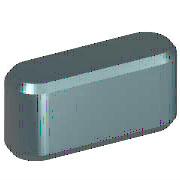
# Autodesk Inventor part: 键 GB/T 1566 A14 x 6 x 40
Saved by Autodesk Inventor 2025 (Build 290162000, 162)
## iProperties
Created: 2024-01-20
Part Number: 键 GB/T 1566 A14 x 6 x 40
Material: 钢，软
Description: 方形和矩形窄键槽
Document SubType Name: Modeling
Standard: GB/T 1566-2003
Designer: ASUS
Standard Revision: 2003
Standards Organization: GB
Language: zh-CN
Size Designation: A - 14 x 6 x 40
Categories: <MemberInstance><Categories><Category DisplayName="轴用零件" InternalName="7f7aeb1f-a693-4053-b835-cee3144e0d98" Mnemonic="SHFT"><Category DisplayName="键" InternalName="7048e72f-fdca-4e3b-88b7-55969eb6630e" Mnemonic="KEY"><CategoryParameter DisplayName="宽度" InternalName="34be0dd5-dba5-4911-b4ec-c22f2bfaa692" Mnemonic="kwdth"/><CategoryParameter DisplayName="最大轴肩直径" InternalName="95a81a26-4bdb-43e8-b886-6e2d08494928" Mnemonic="maxshdia"/><CategoryParameter DisplayName="最小轴肩直径" InternalName="b06394f3-cee7-4e5b-902c-663fb38acff4" Mnemonic="minshdia"/><CategoryParameter DisplayName="尺寸" InternalName="da4729c0-75a4-4053-9158-804a4a937d72" Mnemonic="keysize"/><CategoryParameter DisplayName="轴直径范围 (最小 - 最大)" InternalName="e5432c95-44d4-4c4b-a96d-eed0500887aa" Mnemonic="shaftdiarng"/><CategoryParameter DisplayName="轴直径" InternalName="ff971ec2-6a20-455a-900e-83f11d6bc337" Mnemonic="shaftdia"/><Category DisplayName="键 - 机制" InternalName="7a219f9c-bd0a-4811-91fb-2e47d97adffa" Mnemonic="PRLKEY"><CategoryParameter DisplayName="类型" InternalName="16552a72-3a79-47b2-9cce-0bdb5ab712ec" Mnemonic="keytype"/><CategoryParameter DisplayName="长度" InternalName="2aaf8abc-e798-4f7a-b8d4-83df963ddd80" Mnemonic="klen"/><CategoryParameter DisplayName="平键槽深" InternalName="b2aecbbc-9c00-4ee8-a417-d7ce8bca5723" Mnemonic="groovedepth"/><CategoryParameter DisplayName="高度" InternalName="d0342fb0-ff3c-42cf-83d6-cbe58e85d3e8" Mnemonic="kheig"/><CategoryParameter DisplayName="键槽深" InternalName="e370d4da-8754-4912-963a-6e35f2b6573a" Mnemonic="hubdepth"/><Category DisplayName="圆形" InternalName="c65a28b4-1924-4107-97a1-2d8922e9707a" Mnemonic="PRLKEYROUND"/></Category></Category></Category><Category DisplayName="数据类型" InternalName="23b78d0f-2648-40c6-8793-ca6db495c9e8" Mnemonic="DATATYPE"><CategoryParameter DisplayName="显示名" InternalName="05415f3d-3907-474b-a020-eb9d644f4cf3" Mnemonic="DISPLAYNAME"/><CategoryParameter DisplayName="标准" InternalName="0c0a119c-1e12-4c84-803f-101930972f5e" Mnemonic="STANDARD"/><CategoryParameter DisplayName="描述" InternalName="13903e3d-64b1-4950-80da-f627842ea37f" Mnemonic="DESCRIPTION"/><CategoryParameter DisplayName="规格" InternalName="2675968c-4ce5-49e0-a4f5-552d29089031" Mnemonic="DESIGNATION"/><CategoryParameter DisplayName="默认列" InternalName="2af9ec52-faaa-4026-b378-f9fa4afca842" Mnemonic="DEFAULTROW"/><CategoryParameter DisplayName="文件夹名称" InternalName="3f06958e-8713-4116-9be7-ed6184ecc97b" Mnemonic="FOLDERNAME"/><CategoryParameter DisplayName="版本指南" InternalName="45a75005-10b1-4dfc-8d6d-dfe629f0b93c" Mnemonic="REVISIONGUID"/><CategoryParameter DisplayName="文件名" InternalName="8b46a4cc-9585-4fed-90c3-899f57e09a73" Mnemonic="FILENAME"/><CategoryParameter DisplayName="标准组织" InternalName="8f5914e1-4693-403f-8ab5-d37768198c9d" Mnemonic="STDSORG"/><CategoryParameter DisplayName="系列版本" InternalName="914462f6-6e19-4b14-ba84-155b9680b1d0" Mnemonic="FAMILYREVISION"/><CategoryParameter DisplayName="标准版本" InternalName="91d5a463-65c2-4fde-b823-3b7fea5e8e17" Mnemonic="STANDARDREVISION"/><CategoryParameter DisplayName="成员版本" InternalName="a65d44b9-392f-4f4f-857b-e4b3d54996fe" Mnemonic="MEMBERREVISION"/><CategoryParameter DisplayName="剪裁格式" InternalName="bc51e27b-3422-4e78-93ef-cec197ddf230" Mnemonic="CLIPFORMAT"/><CategoryParameter DisplayName="制造商" InternalName="cd6c7a72-a28a-4e50-99a9-2c7f4e13e5ad" Mnemonic="MANUFACTURER"/><CategoryParameter DisplayName="内部名称" InternalName="cf1d0246-76d9-4b4a-8305-fa0409afb5c1" Mnemonic="INTERNALNAME"/><CategoryParameter DisplayName="是否公制" InternalName="e2385c5b-1ea4-4823-96a8-8de651266ec3" Mnemonic="ISMETRIC"/><Category DisplayName="零件" InternalName="c0e0b642-3bcb-4cc8-9e80-f96d35c4afa4" Mnemonic="PART"><CategoryParameter DisplayName="零件代号" InternalName="016b6077-bfbe-49bd-92c9-d8d59c39c941" Mnemonic="PARTNUMBER"/><CategoryParameter DisplayName="库存编号" InternalName="4dba7c1c-e26c-444e-836c-b08b433409a8" Mnemonic="STOCKNUMBER"/><CategoryParameter DisplayName="材料键" InternalName="5c9a8adb-dd2b-4535-b97f-0a94a95fe41f" Mnemonic="MATERIALKEY"/><CategoryParameter DisplayName="材料" InternalName="818a152a-d3c3-49ca-80ee-df7d91421b8e" Mnemonic="MATERIAL"/></Category></Category><Category DisplayName="先前版本映射" InternalName="cd87c42b-3e48-431e-b5c0-1cbeb14dfe77" Mnemonic="LEGACYMAP"><CategoryParameter DisplayName="唯一 DA 成员 ID" InternalName="0918ad47-427f-4fed-ae26-24c81c58f590" Mnemonic="DACOOKIE"/><CategoryParameter DisplayName="合并11 ID" InternalName="0ee8fb18-e2ed-4f39-96f6-1f4b5f50aa71" Mnemonic="MERGE11"/><CategoryParameter DisplayName="唯一 CC 成员 ID" InternalName="5193edd4-b2b0-4ab4-9d54-de900eee34e0" Mnemonic="CCCOOKIE"/><CategoryParameter DisplayName="分割 ID" InternalName="72b5c83c-be7f-45c4-ae51-9160ea6deb26" Mnemonic="SPLIT"/><CategoryParameter DisplayName="成员 ID" InternalName="8e5e0294-fc51-4c8f-b3d7-003dc5ed94f6" Mnemonic="MEMBERID"/><CategoryParameter DisplayName="目录名" InternalName="d99d1e27-aa94-4de2-af4c-c348882a6f4f" Mnemonic="CATALOGNAME"/><CategoryParameter DisplayName="系列编号" InternalName="e705e1f4-09cb-413e-91f9-551b4188271e" Mnemonic="FAMILYNUMBER"/></Category></Categories><FamilyTemplate Id="si0114"><FamilyTemplateParameters><FamilyTemplateParameter ObjectType="kUserParameterObject" ValueType="xs:double" Id="1" ObjectReferenceKey="NLG"/><FamilyTemplateParameter ObjectType="kUserParameterObject" ValueType="xs:double" Id="2" ObjectReferenceKey="WDMIN"/><FamilyTemplateParameter ObjectType="kUserParameterObject" ValueType="xs:double" Id="3" ObjectReferenceKey="PH"/><FamilyTemplateParameter ObjectType="kUserParameterObject" ValueType="xs:double" Id="4" ObjectReferenceKey="PHH"/><FamilyTemplateParameter ObjectType="kUserParameterObject" ValueType="xs:double" Id="5" ObjectReferenceKey="PLB2"/><FamilyTemplateParameter ObjectType="kUserParameterObject" ValueType="xs:double" Id="6" ObjectReferenceKey="PNT"/><FamilyTemplateParameter ObjectType="kUserParameterObject" ValueType="xs:double" Id="7" ObjectReferenceKey="WDMAX"/><FamilyTemplateParameter ObjectType="kUserParameterObject" ValueType="xs:double" Id="8" ObjectReferenceKey="PLB1"/><FamilyTemplateParameter ObjectType="kUserParameterObject" ValueType="xs:double" Id="9" ObjectReferenceKey="PB"/><FamilyTemplateParameter ObjectType="kUserParameterObject" ValueType="xs:double" Id="10" ObjectReferenceKey="RR"/><FamilyTemplateParameter ObjectType="kUserParameterObject" ValueType="xs:double" Id="11" ObjectReferenceKey="PUEB"/><FamilyTemplateParameter ObjectType="kPropertyObject" ValueType="xs:string" Id="100" ObjectReferenceKey="{32853F0F-3444-11d1-9E93-0060B03C1CA6}" SubObjectId="52"/><FamilyTemplateParameter ObjectType="kPropertyObject" ValueType="xs:string" Id="105" ObjectReferenceKey="{32853F0F-3444-11d1-9E93-0060B03C1CA6}" SubObjectId="5"/><FamilyTemplateParameter ObjectType="kPartComponentDefinitionObject" ValueType="xs:string" Id="110" SubObjectId="Material"/></FamilyTemplateParameters></FamilyTemplate><CategoryParameterMap><ParamToTemplateMap><ParamToTemplate CategoryParameter="//CategoryParameter[@InternalName='05415f3d-3907-474b-a020-eb9d644f4cf3']" ConstantValue="Key GB/T 1566-2003 Type A"/><ParamToTemplate CategoryParameter="//CategoryParameter[@InternalName='cf1d0246-76d9-4b4a-8305-fa0409afb5c1']" ConstantValue="77fd1fdf-4ae4-4465-aad0-a3ecc73b3757"/><ParamToTemplate CategoryParameter="//CategoryParameter[@InternalName='3f06958e-8713-4116-9be7-ed6184ecc97b']" ConstantValue="GB_T 1566-2003 A"/><ParamToTemplate CategoryParameter="//CategoryParameter[@InternalName='914462f6-6e19-4b14-ba84-155b9680b1d0']" ConstantValue="10"/><ParamToTemplate CategoryParameter="//CategoryParameter[@InternalName='bc51e27b-3422-4e78-93ef-cec197ddf230']" ConstantValue="CF_INVENTOR.STDPARTS"/><ParamToTemplate CategoryParameter="//CategoryParameter[@InternalName='e2385c5b-1ea4-4823-96a8-8de651266ec3']" ConstantValue="true"/><ParamToTemplate CategoryParameter="//CategoryParameter[@InternalName='13903e3d-64b1-4950-80da-f627842ea37f']" ConstantValue="Square and rectangular thin keyways"/><ParamToTemplate CategoryParameter="//CategoryParameter[@InternalName='8f5914e1-4693-403f-8ab5-d37768198c9d']" ConstantValue="GB"/><ParamToTemplate CategoryParameter="//CategoryParameter[@InternalName='0c0a119c-1e12-4c84-803f-101930972f5e']" ConstantValue="GB/T 1566-2003"/><ParamToTemplate CategoryParameter="//CategoryParameter[@InternalName='cd6c7a72-a28a-4e50-99a9-2c7f4e13e5ad']" TemplateParameter="104"/><ParamToTemplate CategoryParameter="//CategoryParameter[@InternalName='91d5a463-65c2-4fde-b823-3b7fea5e8e17']" ConstantValue="2003"/><ParamToTemplate CategoryParameter="//CategoryParameter[@InternalName='45a75005-10b1-4dfc-8d6d-dfe629f0b93c']" ConstantValue="51c6a18e-fa1a-4ca6-9ff8-233106514174"/><ParamToTemplate CategoryParameter="//CategoryParameter[@InternalName='2af9ec52-faaa-4026-b378-f9fa4afca842']" ConstantValue="10"/><ParamToTemplate CategoryParameter="//CategoryParameter[@InternalName='d99d1e27-aa94-4de2-af4c-c348882a6f4f']" ConstantValue="GB"/><ParamToTemplate CategoryParameter="//CategoryParameter[@InternalName='e705e1f4-09cb-413e-91f9-551b4188271e']" ConstantValue="295"/><ParamToTemplate CategoryParameter="//CategoryParameter[@InternalName='8b46a4cc-9585-4fed-90c3-899f57e09a73']" ConstantValue="键 GB/T 1566 A14 x 6 x 40"/><ParamToTemplate CategoryParameter="//CategoryParameter[@InternalName='a65d44b9-392f-4f4f-857b-e4b3d54996fe']" ConstantValue="C2D96F29-4DB2-4EBC-AAA9-F59C0D21B4C7"/><ParamToTemplate CategoryParameter="//CategoryParameter[@InternalName='e5432c95-44d4-4c4b-a96d-eed0500887aa']" ConstantValue="44 - 50"/><ParamToTemplate CategoryParameter="//CategoryParameter[@InternalName='da4729c0-75a4-4053-9158-804a4a937d72']" ConstantValue="14x6"/><ParamToTemplate CategoryParameter="//CategoryParameter[@InternalName='16552a72-3a79-47b2-9cce-0bdb5ab712ec']" ConstantValue="A"/><ParamToTemplate CategoryParameter="//CategoryParameter[@InternalName='8e5e0294-fc51-4c8f-b3d7-003dc5ed94f6']" ConstantValue="770"/><ParamToTemplate CategoryParameter="//CategoryParameter[@InternalName='2675968c-4ce5-49e0-a4f5-552d29089031']" TemplateParameter="100"/><ParamToTemplate CategoryParameter="//CategoryParameter[@InternalName='818a152a-d3c3-49ca-80ee-df7d91421b8e']" TemplateParameter="110"/><ParamToTemplate CategoryParameter="//CategoryParameter[@InternalName='2aaf8abc-e798-4f7a-b8d4-83df963ddd80']" TemplateParameter="1"/><ParamToTemplate CategoryParameter="//CategoryParameter[@InternalName='016b6077-bfbe-49bd-92c9-d8d59c39c941']" TemplateParameter="105"/><ParamToTemplate CategoryParameter="//CategoryParameter[@InternalName='34be0dd5-dba5-4911-b4ec-c22f2bfaa692']" TemplateParameter="9"/><ParamToTemplate CategoryParameter="//CategoryParameter[@InternalName='d0342fb0-ff3c-42cf-83d6-cbe58e85d3e8']" TemplateParameter="3"/><ParamToTemplate CategoryParameter="//CategoryParameter[@InternalName='b2aecbbc-9c00-4ee8-a417-d7ce8bca5723']" TemplateParameter="6"/><ParamToTemplate CategoryParameter="//CategoryParameter[@InternalName='e370d4da-8754-4912-963a-6e35f2b6573a']" TemplateParameter="11"/><ParamToTemplate CategoryParameter="//CategoryParameter[@InternalName='95a81a26-4bdb-43e8-b886-6e2d08494928']" TemplateParameter="7"/><ParamToTemplate CategoryParameter="//CategoryParameter[@InternalName='b06394f3-cee7-4e5b-902c-663fb38acff4']" TemplateParameter="2"/></ParamToTemplateMap></CategoryParameterMap></MemberInstance>
Density: 7.85 g/cm^3
Appearance: 半抛光
IsCustomPart: 0
Author: ASUS
Autodesk Inventor part; units mm, degrees
sketch "草图1" plane through (0, 0, 0) normal (0, 0, 1) x (1, 0, 0)
  line L0 (7, 7) -> (33, 7)
  line L1 (33, -7) -> (7, -7)
  arc A0 (7, 7) -> (7, -7) centre (7, 0) ccw
  line L2 (0, 9.4) -> (0, -7.4) projected
  line L3 (-5, 0) -> (30, 0) projected
  arc A1 (33, -7) -> (33, 7) centre (33, 0) ccw
  line L4 (40, 0) -> (40, 7) construction
  dimension "d0" = 7
  dimension "d13" = 7
  dimension "d14" = 40
  constraints: 6 end point, 5 point on circle, 4 tangent, 3 point on line, 2 centre point, 1 horizontal, 1 parallel, 1 perpendicular
  measures "d0" radius of A0
  measures "d13" radius of A1
  measures "d14" distance between parallel lines of L4 L2
ref_plane "Work Plane1" through (0, 0, -3.5) normal (0, 0, 1) x (1, 0, 0)
ref_plane "Work Plane2" through (0, 0, 2.5) normal (0, 0, 1) x (1, 0, 0)
extrude "轴承体1" add sketch "草图1" against normal up to surface (6 mm away) from surface at 2.5
chamfer "倒角1" distance 0.6 angle 45 6 edges at (0, 0, 2.5) (20, 7, 2.5) (20, -7, 2.5) (0, 0, -3.5) (20, 7, -3.5) (20, -7, -3.5)
ref_plane "Work Plane3" through (40, 0, -2.9) normal (1, 0, 0) x (0, 1, 0)
equation "\"d0\" = 0.5 * PB"
equation "\"d13\" = 0.5 * PB"
equation "\"d14\" = NLG"
equation "\"d8\" = PHH"
equation "\"d9\" = PHH"
equation "\"d1\" = -PNT"
equation "\"d2\" = PH - PNT"
equation "\"NLG\" = 40"
equation "\"PB\" = 14"
equation "\"PNT\" = 3.5"
equation "\"PH\" = 6"
equation "\"PHH\" = 0.6"
equation "\"WDMIN\" = 44"
equation "\"RR\" = 0.25"
equation "\"PUEB\" = 2.8"
body "Solid1"
